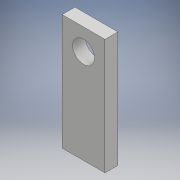
# Autodesk Inventor part: Raket_Arme_Motor
Saved by Autodesk Inventor 2018 (Build 220112000, 112)
## iProperties
Created: 2017-08-14
Part Number: Raket_Arme_Motor
Material: Generic
Document SubType Name: Modeling
Designer: andre
Density: 1 g/cm^3
Appearance: Default
Author: andre
## iProperties of the stored document Raket_Arme_Motor_3DPrint.ipt
Created: 2017-08-14
Part Number: Raket_Arme_Motor_3DPrint
Material: Generic
Document SubType Name: Modeling
Designer: andre
Density: 1 g/cm^3
Appearance: Default
Author: andre
Autodesk Inventor part; units mm, degrees
ref_plane "YZ Plane" through (0, 0, 0) normal (1, 0, 0) x (0, 1, 0)
ref_plane "XZ Plane" through (0, 0, 0) normal (0, 1, 0) x (-1, 0, 0)
ref_plane "XY Plane" through (0, 0, 0) normal (0, 0, 1) x (1, 0, 0)
sketch "Sketch1" plane through (0, 0, 0) normal (0, 1, 0) x (-1, 0, 0)
  line L0 (0, 0) -> (10, 0)
  line L1 (10, 0) -> (10, -27)
  line L2 (10, -27) -> (0, -27)
  line L3 (0, -27) -> (0, 0)
  dimension "d0" = 10
  dimension "d1" = 27
  constraints: 8 end point, 2 parallel, 1 horizontal, 1 perpendicular
  measures "d0" distance of L1.end L2.end
  measures "d1" distance of L0.end L1.end
extrude "Extrusion1" add sketch "Sketch1" along normal blind 10
sketch "Sketch2" plane through (0, 10, 0) normal (0, 1, 0) x (1, 0, 0)
  line L0 (-10, 27) -> (-10, 0) projected
  line L1 (-10, 0) -> (-10, 5)
  circle A0 centre (-5, 5) radius 2.55
  point P0 (0, 0)
  dimension "d4" = 5
  dimension "d5" = 5.1
  constraints: 2 end point, 1 centre point, 1 point on line
  measures "d4" distance of L0.end L1.end
  measures "d5" diameter of A0
extrude "Extrusion2" cut sketch "Sketch2" against normal blind 10
sketch "Sketch4" plane through (0, 10, 0) normal (0, 1, 0) x (1, 0, 0)
  line L0 (0, 27) -> (-10, 27) projected
  line L1 (-10, 27) -> (-10, 0) projected
  line L2 (0, 27) -> (-10, 27)
  line L3 (-10, 27) -> (-10, 0)
  line L4 (-10, 0) -> (0, 0)
  line L5 (0, 0) -> (0, 27)
  point P0 (0, 0)
  dimension "d13" = 27
  constraints: 8 end point, 2 parallel, 1 horizontal, 1 perpendicular, 1 point on line
  measures "d13" distance of L3.end L2.end
extrude "Extrusion4" cut sketch "Sketch4" against normal blind 7
body "Solid1"
